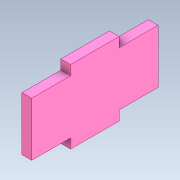
# Autodesk Inventor part: FrontWall
Saved by Autodesk Inventor 2021 (Build 250183000, 183)
## iProperties
Created: 2021-08-31
Part Number: FrontWall
Material: ABS Plastic
Document SubType Name: Modeling
Designer: digge
Density: 1.06 g/cm^3
Appearance: Pink
Author: digge
Autodesk Inventor part; units mm, degrees
ref_plane "YZ Plane" through (0, 0, 0) normal (1, 0, 0) x (0, 1, 0)
ref_plane "XZ Plane" through (0, 0, 0) normal (0, 1, 0) x (-1, 0, 0)
ref_plane "XY Plane" through (0, 0, 0) normal (0, 0, 1) x (1, 0, 0)
sketch "Sketch1" plane through (0, 0, 0) normal (1, 0, 0) x (0, 1, 0)
  line L0 (108.4, 213) -> (53, 213)
  line L1 (53, 213) -> (53, 173)
  line L2 (53, 173) -> (43, 173)
  line L3 (43, 173) -> (43, 123)
  line L4 (43, 123) -> (53, 123)
  line L5 (53, 123) -> (53, 83)
  line L6 (53, 83) -> (108.4, 83)
  line L7 (108.4, 83) -> (108.4, 123)
  line L8 (108.4, 123) -> (118.4, 123)
  line L9 (118.4, 123) -> (118.4, 173)
  line L10 (118.4, 173) -> (108.4, 173)
  line L11 (108.4, 213) -> (108.4, 173)
  line L12 (43, 148) -> (118.4, 148) construction
  point P0 (0, 0)
  dimension "d0" = 10
  dimension "d1" = 10
  dimension "d2" = 50
  dimension "d3" = 55.4
  dimension "d4" = 130
  constraints: 26 end point, 8 perpendicular, 6 point on line, 2 midpoint, 1 horizontal, 1 other
  measures "d0" distance of L1.end L2.end
  measures "d1" distance of L9.end L10.end
  measures "d2" distance of L8.end L9.end
  measures "d3" distance of L0.start L0.end
  measures "d4" distance between parallel lines of L6 L0
extrude "Extrusion1" add sketch "Sketch1" along normal blind 10
equation "\"d0\" = Width"
equation "\"d1\" = Width"
equation "\"d5\" = Width"
equation "\"Width\" = 10"
body "Solid1"
